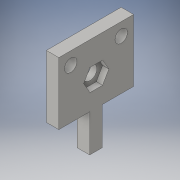
# Autodesk Inventor part: Holder
Saved by Autodesk Inventor 2016 (Build 200138000, 138)
## iProperties
Created: 2016-04-23
Part Number: Holder
Material: Generic
Document SubType Name: Modeling
Designer: rubenjm
Density: 1 g/cm^3
Appearance: Default
Author: rubenjm
Autodesk Inventor part; units mm, degrees
ref_plane "YZ Plane" through (0, 0, 0) normal (1, 0, 0) x (0, 1, 0)
ref_plane "XZ Plane" through (0, 0, 0) normal (0, 1, 0) x (-1, 0, 0)
ref_plane "XY Plane" through (0, 0, 0) normal (0, 0, 1) x (1, 0, 0)
sketch "Sketch1" plane through (0, 0, 0) normal (1, 0, 0) x (0, 1, 0)
  circle A0 centre (27.2595, -37.4781) radius 6.985 construction
  circle A1 centre (50.8, -12.0577) radius 6.35
  line L0 (63.5, 0) -> (50.8, 0) construction
  line L1 (50.8, 0) -> (50.8, -12.7) construction
  line L2 (50.8, -12.7) -> (63.5, -12.7) construction
  line L3 (63.5, -12.7) -> (63.5, 0) construction
  circle A2 centre (50.8, -63.5) radius 6.35
  line L4 (16.147, -31.0623) -> (27.2595, -24.6465) construction
  line L5 (27.2595, -24.6465) -> (38.372, -31.0623) construction
  line L6 (38.372, -31.0623) -> (38.372, -43.8939) construction
  line L7 (38.372, -43.8939) -> (27.2595, -50.3097) construction
  line L8 (27.2595, -50.3097) -> (16.147, -43.8939) construction
  line L9 (16.147, -43.8939) -> (16.147, -31.0623) construction
  line L10 (0, -31.4288) -> (-38.1, -31.4288)
  line L11 (-38.1, -31.4288) -> (-38.1, -44.1288)
  line L12 (-38.1, -44.1288) -> (0, -44.1288)
  line L13 (63.5, 0) -> (0, 0)
  line L14 (0, -76.2) -> (63.5, -76.2)
  line L15 (63.5, -76.2) -> (63.5, 0)
  line L16 (0, 0) -> (0, -31.4288)
  line L17 (0, -44.1288) -> (0, -76.2)
  dimension "d9" = 13.97
  dimension "d12" = 12.7
  dimension "d13" = 12.7
  dimension "d18" = 22.225
  dimension "d21" = 38.1
  dimension "d22" = 12.7
  dimension "d23" = 63.5
  dimension "d24" = 76.2
  dimension "d38" = 38.1
  constraints: 36 end point, 6 parallel, 4 perpendicular, 3 centre point, 3 horizontal, 1 coincident, 13 other
  measures "d9" diameter of A0
  measures "d12" diameter of A1
  measures "d13" distance of L2.end L1.end
  measures "d18" distance between parallel lines of L9 L6
  measures "d21" distance of L12.end L11.end
  measures "d22" distance of L11.end L10.end
  measures "d23" distance of L14.end L14.start
  measures "d24" distance of L14.start L13.end
  measures "d38" distance of L10.start L10.end
extrude "Extrusion3" add sketch "Sketch1" along normal blind 12.7
sketch "Sketch2" plane through (12.7, 0, 0) normal (1, 0, 0) x (0, 0, -1)
  line L0 (0, 0) -> (38.1, 0) construction
  line L1 (38.1, 0) -> (38.1, 27.94) construction
  line L2 (31.6842, 16.8275) -> (25.2684, 27.94)
  line L3 (25.2684, 27.94) -> (31.6842, 39.0525)
  line L4 (31.6842, 39.0525) -> (44.5158, 39.0525)
  line L5 (44.5158, 39.0525) -> (50.9316, 27.94)
  line L6 (50.9316, 27.94) -> (44.5158, 16.8275)
  line L7 (44.5158, 16.8275) -> (31.6842, 16.8275)
  point P0 (38.1, 16.8275)
  dimension "d29" = 38.1
  dimension "d30" = 27.94
  dimension "d31" = 90
  dimension "d32" = 22.225
  constraints: 16 end point, 1 coincident, 1 horizontal, 1 midpoint, 1 perpendicular, 1 point on line, 13 other
  measures "d29" distance of L0.start L0.end
  measures "d30" distance of L0.end L1.end
  measures "d31" angle of L1 L0
  measures "d32" distance between parallel lines of L7 L4
extrude "Extrusion4" cut sketch "Sketch2" against normal blind 6.35
sketch "Sketch3" plane through (6.35, 0, 0) normal (1, 0, 0) x (0, 0, -1)
  line L0 (25.2684, 27.94) -> (31.6842, 39.0525) construction
  line L1 (31.6842, 39.0525) -> (44.5158, 16.8275) construction
  circle A0 centre (38.1, 27.94) radius 6.985
  point P0 (0, 0)
  dimension "d35" = 13.97
  constraints: 2 end point, 1 centre point, 1 midpoint
  measures "d35" diameter of A0
extrude "Extrusion5" cut sketch "Sketch3" along normal through all both and the other way through all
equation "\"d38\" = d21"
body "Solid3"
